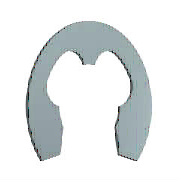
# Autodesk Inventor part: JIS B 2804 E - 3
Saved by Autodesk Inventor 2017 (Build 210142000, 142)
## iProperties
Created: 2016-02-22
Part Number: JIS B 2804 E - 3
Material: Acier, doux
Description: Rondelle élastique d´arrêt
Document SubType Name: Modeling
Standard: JIS B 2804
Designer: Adrien MARY
Standard Revision: 2010
Standards Organization: JIS
Language: fr-FR
Size Designation: 3
Categories: <MemberInstance><Categories><Category DisplayName="Pièces d'arbre" InternalName="7f7aeb1f-a693-4053-b835-cee3144e0d98" Mnemonic="SHFT"><Category DisplayName="Anneaux élastiques" InternalName="413b042a-1f46-4051-a560-0e0e417af91f" Mnemonic="CLIP"><CategoryParameter DisplayName="Epaisseur" InternalName="230c7f7c-2544-4c6d-b8d5-773e831b23fa" Mnemonic="thick"/><CategoryParameter DisplayName="Diamètre de rainure" InternalName="4054b45c-161d-4ad6-befb-f30b3855ce84" Mnemonic="grvdia"/><CategoryParameter DisplayName="Largeur de rainure" InternalName="4dde6996-4bf1-443b-8317-d4f4fc6b9be0" Mnemonic="NB"/><CategoryParameter DisplayName="Diamètre d'arbe" InternalName="a433c9ab-b9eb-4798-a453-f2210a67728e" Mnemonic="shaftdia"/><Category DisplayName="Externe" InternalName="a9a2b132-a8be-48ab-9c3d-0c324a909558" Mnemonic="OUCLIP"><CategoryParameter DisplayName="Diamètre min. d'arbre" InternalName="62b77b9b-1e86-4b9a-9911-d7c0fa48fc9a" Mnemonic="shaftdiamin"/><CategoryParameter DisplayName="Diamètre extérieur" InternalName="a3599e7b-be7c-41b5-9a50-6dab253b0906" Mnemonic="outdia"/></Category></Category></Category><Category DisplayName="Type de données" InternalName="23b78d0f-2648-40c6-8793-ca6db495c9e8" Mnemonic="DATATYPE"><CategoryParameter DisplayName="AfficherNom" InternalName="05415f3d-3907-474b-a020-eb9d644f4cf3" Mnemonic="DISPLAYNAME"/><CategoryParameter DisplayName="Norme" InternalName="0c0a119c-1e12-4c84-803f-101930972f5e" Mnemonic="STANDARD"/><CategoryParameter DisplayName="Description" InternalName="13903e3d-64b1-4950-80da-f627842ea37f" Mnemonic="DESCRIPTION"/><CategoryParameter DisplayName="Désignation" InternalName="2675968c-4ce5-49e0-a4f5-552d29089031" Mnemonic="DESIGNATION"/><CategoryParameter DisplayName="Ligne par défaut" InternalName="2af9ec52-faaa-4026-b378-f9fa4afca842" Mnemonic="DEFAULTROW"/><CategoryParameter DisplayName="Nom de dossier" InternalName="3f06958e-8713-4116-9be7-ed6184ecc97b" Mnemonic="FOLDERNAME"/><CategoryParameter DisplayName="Guide révision" InternalName="45a75005-10b1-4dfc-8d6d-dfe629f0b93c" Mnemonic="REVISIONGUID"/><CategoryParameter DisplayName="NomFichier" InternalName="8b46a4cc-9585-4fed-90c3-899f57e09a73" Mnemonic="FILENAME"/><CategoryParameter DisplayName="OrgNorm" InternalName="8f5914e1-4693-403f-8ab5-d37768198c9d" Mnemonic="STDSORG"/><CategoryParameter DisplayName="Version de la famille" InternalName="914462f6-6e19-4b14-ba84-155b9680b1d0" Mnemonic="FAMILYREVISION"/><CategoryParameter DisplayName="Version standard" InternalName="91d5a463-65c2-4fde-b823-3b7fea5e8e17" Mnemonic="STANDARDREVISION"/><CategoryParameter DisplayName="Révision de membre" InternalName="a65d44b9-392f-4f4f-857b-e4b3d54996fe" Mnemonic="MEMBERREVISION"/><CategoryParameter DisplayName="DélimiterFormat" InternalName="bc51e27b-3422-4e78-93ef-cec197ddf230" Mnemonic="CLIPFORMAT"/><CategoryParameter DisplayName="Fabricant" InternalName="cd6c7a72-a28a-4e50-99a9-2c7f4e13e5ad" Mnemonic="MANUFACTURER"/><CategoryParameter DisplayName="NomInterne" InternalName="cf1d0246-76d9-4b4a-8305-fa0409afb5c1" Mnemonic="INTERNALNAME"/><CategoryParameter DisplayName="Métrique" InternalName="e2385c5b-1ea4-4823-96a8-8de651266ec3" Mnemonic="ISMETRIC"/><Category DisplayName="Pièce" InternalName="c0e0b642-3bcb-4cc8-9e80-f96d35c4afa4" Mnemonic="PART"><CategoryParameter DisplayName="Numéro de pièce" InternalName="016b6077-bfbe-49bd-92c9-d8d59c39c941" Mnemonic="PARTNUMBER"/><CategoryParameter DisplayName="Numéro de stock" InternalName="4dba7c1c-e26c-444e-836c-b08b433409a8" Mnemonic="STOCKNUMBER"/><CategoryParameter DisplayName="Clé matière" InternalName="5c9a8adb-dd2b-4535-b97f-0a94a95fe41f" Mnemonic="MATERIALKEY"/><CategoryParameter DisplayName="Matière" InternalName="818a152a-d3c3-49ca-80ee-df7d91421b8e" Mnemonic="MATERIAL"/></Category></Category><Category DisplayName="CarteHéritée" InternalName="cd87c42b-3e48-431e-b5c0-1cbeb14dfe77" Mnemonic="LEGACYMAP"><CategoryParameter DisplayName="ID membre DA unique" InternalName="0918ad47-427f-4fed-ae26-24c81c58f590" Mnemonic="DACOOKIE"/><CategoryParameter DisplayName="ID de fusion11" InternalName="0ee8fb18-e2ed-4f39-96f6-1f4b5f50aa71" Mnemonic="MERGE11"/><CategoryParameter DisplayName="ID membre CC unique" InternalName="5193edd4-b2b0-4ab4-9d54-de900eee34e0" Mnemonic="CCCOOKIE"/><CategoryParameter DisplayName="ID de division" InternalName="72b5c83c-be7f-45c4-ae51-9160ea6deb26" Mnemonic="SPLIT"/><CategoryParameter DisplayName="IDMembre" InternalName="8e5e0294-fc51-4c8f-b3d7-003dc5ed94f6" Mnemonic="MEMBERID"/><CategoryParameter DisplayName="NomCatologue" InternalName="d99d1e27-aa94-4de2-af4c-c348882a6f4f" Mnemonic="CATALOGNAME"/><CategoryParameter DisplayName="NuméroFamille" InternalName="e705e1f4-09cb-413e-91f9-551b4188271e" Mnemonic="FAMILYNUMBER"/></Category></Categories><FamilyTemplate Id="si0132"><FamilyTemplateParameters><FamilyTemplateParameter ObjectType="kUserParameterObject" ValueType="xs:double" Id="1" ObjectReferenceKey="WDMIN"/><FamilyTemplateParameter ObjectType="kUserParameterObject" ValueType="xs:double" Id="2" ObjectReferenceKey="SNB"/><FamilyTemplateParameter ObjectType="kUserParameterObject" ValueType="xs:double" Id="3" ObjectReferenceKey="SD2"/><FamilyTemplateParameter ObjectType="kUserParameterObject" ValueType="xs:double" Id="4" ObjectReferenceKey="SD"/><FamilyTemplateParameter ObjectType="kUserParameterObject" ValueType="xs:double" Id="5" ObjectReferenceKey="ND"/><FamilyTemplateParameter ObjectType="kUserParameterObject" ValueType="xs:double" Id="6" ObjectReferenceKey="WDMAX"/><FamilyTemplateParameter ObjectType="kUserParameterObject" ValueType="xs:double" Id="7" ObjectReferenceKey="BUBRMI"/><FamilyTemplateParameter ObjectType="kUserParameterObject" ValueType="xs:double" Id="8" ObjectReferenceKey="WD"/><FamilyTemplateParameter ObjectType="kUserParameterObject" ValueType="xs:double" Id="9" ObjectReferenceKey="NND"/><FamilyTemplateParameter ObjectType="kPropertyObject" ValueType="xs:string" Id="100" ObjectReferenceKey="{32853F0F-3444-11d1-9E93-0060B03C1CA6}" SubObjectId="52"/><FamilyTemplateParameter ObjectType="kPropertyObject" ValueType="xs:string" Id="105" ObjectReferenceKey="{32853F0F-3444-11d1-9E93-0060B03C1CA6}" SubObjectId="5"/><FamilyTemplateParameter ObjectType="kPartComponentDefinitionObject" ValueType="xs:string" Id="110" SubObjectId="Material"/></FamilyTemplateParameters></FamilyTemplate><CategoryParameterMap><ParamToTemplateMap><ParamToTemplate CategoryParameter="//CategoryParameter[@InternalName='05415f3d-3907-474b-a020-eb9d644f4cf3']" ConstantValue="JIS B 2804 E"/><ParamToTemplate CategoryParameter="//CategoryParameter[@InternalName='cf1d0246-76d9-4b4a-8305-fa0409afb5c1']" ConstantValue="B983131E-6E8A-4140-85C7-FDB04EB2BDA0"/><ParamToTemplate CategoryParameter="//CategoryParameter[@InternalName='3f06958e-8713-4116-9be7-ed6184ecc97b']" ConstantValue="JIS B 2804 E"/><ParamToTemplate CategoryParameter="//CategoryParameter[@InternalName='914462f6-6e19-4b14-ba84-155b9680b1d0']" ConstantValue="10"/><ParamToTemplate CategoryParameter="//CategoryParameter[@InternalName='bc51e27b-3422-4e78-93ef-cec197ddf230']" ConstantValue="CF_INVENTOR.STDPARTS"/><ParamToTemplate CategoryParameter="//CategoryParameter[@InternalName='e2385c5b-1ea4-4823-96a8-8de651266ec3']" ConstantValue="true"/><ParamToTemplate CategoryParameter="//CategoryParameter[@InternalName='13903e3d-64b1-4950-80da-f627842ea37f']" ConstantValue="Spring Retaining Ring"/><ParamToTemplate CategoryParameter="//CategoryParameter[@InternalName='8f5914e1-4693-403f-8ab5-d37768198c9d']" ConstantValue="JIS"/><ParamToTemplate CategoryParameter="//CategoryParameter[@InternalName='0c0a119c-1e12-4c84-803f-101930972f5e']" ConstantValue="JIS B 2804"/><ParamToTemplate CategoryParameter="//CategoryParameter[@InternalName='cd6c7a72-a28a-4e50-99a9-2c7f4e13e5ad']" TemplateParameter="104"/><ParamToTemplate CategoryParameter="//CategoryParameter[@InternalName='91d5a463-65c2-4fde-b823-3b7fea5e8e17']" ConstantValue="2010"/><ParamToTemplate CategoryParameter="//CategoryParameter[@InternalName='45a75005-10b1-4dfc-8d6d-dfe629f0b93c']" ConstantValue="5afb411f-584a-4d28-a564-0e5354a33203"/><ParamToTemplate CategoryParameter="//CategoryParameter[@InternalName='2af9ec52-faaa-4026-b378-f9fa4afca842']" ConstantValue="10"/><ParamToTemplate CategoryParameter="//CategoryParameter[@InternalName='d99d1e27-aa94-4de2-af4c-c348882a6f4f']" ConstantValue="JIS"/><ParamToTemplate CategoryParameter="//CategoryParameter[@InternalName='e705e1f4-09cb-413e-91f9-551b4188271e']" ConstantValue="216"/><ParamToTemplate CategoryParameter="//CategoryParameter[@InternalName='8b46a4cc-9585-4fed-90c3-899f57e09a73']" ConstantValue="JIS B 2804 E - 3 - 5"/><ParamToTemplate CategoryParameter="//CategoryParameter[@InternalName='a65d44b9-392f-4f4f-857b-e4b3d54996fe']" ConstantValue="951B112C-607C-45C7-8E1B-EACF44DB36DB"/><ParamToTemplate CategoryParameter="//CategoryParameter[@InternalName='8e5e0294-fc51-4c8f-b3d7-003dc5ed94f6']" ConstantValue="120"/><ParamToTemplate CategoryParameter="//CategoryParameter[@InternalName='2675968c-4ce5-49e0-a4f5-552d29089031']" TemplateParameter="100"/><ParamToTemplate CategoryParameter="//CategoryParameter[@InternalName='818a152a-d3c3-49ca-80ee-df7d91421b8e']" TemplateParameter="110"/><ParamToTemplate CategoryParameter="//CategoryParameter[@InternalName='4054b45c-161d-4ad6-befb-f30b3855ce84']" TemplateParameter="5"/><ParamToTemplate CategoryParameter="//CategoryParameter[@InternalName='8bbe3f8e-44cf-40a9-a251-3a6edc8168d6']" TemplateParameter="9"/><ParamToTemplate CategoryParameter="//CategoryParameter[@InternalName='016b6077-bfbe-49bd-92c9-d8d59c39c941']" TemplateParameter="105"/><ParamToTemplate CategoryParameter="//CategoryParameter[@InternalName='230c7f7c-2544-4c6d-b8d5-773e831b23fa']" TemplateParameter="4"/><ParamToTemplate CategoryParameter="//CategoryParameter[@InternalName='4dde6996-4bf1-443b-8317-d4f4fc6b9be0']" TemplateParameter="2"/><ParamToTemplate CategoryParameter="//CategoryParameter[@InternalName='a433c9ab-b9eb-4798-a453-f2210a67728e']" TemplateParameter="8"/><ParamToTemplate CategoryParameter="//CategoryParameter[@InternalName='62b77b9b-1e86-4b9a-9911-d7c0fa48fc9a']" TemplateParameter="1"/></ParamToTemplateMap></CategoryParameterMap></MemberInstance>
Density: 7.85 g/cm^3
Appearance: Semi-poli
IsCustomPart: 0
Author: Adrien MARY
Autodesk Inventor part; units mm, degrees
ref_plane "YZ Plane" through (0, 0, 0) normal (1, 0, 0) x (0, 1, 0)
ref_plane "XZ Plane" through (0, 0, 0) normal (0, 1, 0) x (-1, 0, 0)
sketch "Esquisse1" plane through (0, 0, 0) normal (0, 0, 1) x (1, 0, 0)
  circle A0 centre (0, -2.4764) radius 2.5 construction
  line L0 (-0.3, 0.0236) -> (0, 0.0236) construction
  line L1 (-3.206, 0) -> (3.4858, 0) projected
  line L2 (-1.3748, -3.0764) -> (1.3748, -3.0764) construction
  arc A1 (-1.4207, -1.9952) -> (-1.3748, -3.0764) centre (0, -2.4764) ccw
  line L3 (0, 1.949) -> (0, -3.4788) projected
  arc A2 (-0.3, -0.6764) -> (0.3, -0.6764) centre (0, -0.6764) ccw
  arc A3 (2.6558, -4.756) -> (-2.6558, -4.756) centre (0, -2.4764) ccw
  line L4 (-1.8, -1.8764) -> (-1.506, -1.8764)
  line L5 (-0.3, -0.6764) -> (-0.3, -0.3849)
  arc A4 (-0.6, -0.1526) -> (-2.1176, -1.3469) centre (0, -2.4764) ccw
  arc A5 (-0.3, -0.3849) -> (-0.6, -0.1526) centre (-0.54, -0.3849) ccw
  arc A6 (-2.1176, -1.3469) -> (-1.8, -1.8764) centre (-1.8, -1.5164) ccw
  arc A7 (-1.4207, -1.9952) -> (-1.506, -1.8764) centre (-1.506, -1.9664) ccw
  line L6 (0, 1.0236) -> (2.5298, 1.0236) construction
  line L7 (-1.3748, -3.0764) -> (-1.8877, -4.606)
  arc A8 (-2.6558, -4.756) -> (-1.8877, -4.606) centre (-2.3143, -4.4629) ccw
  line L8 (0, -0.9764) -> (-1.2778, -0.9764) construction
  line L9 (1.3748, -3.0764) -> (1.8877, -4.606)
  arc A9 (1.8877, -4.606) -> (2.6558, -4.756) centre (2.3143, -4.4629) ccw
  arc A10 (1.3748, -3.0764) -> (1.4207, -1.9952) centre (0, -2.4764) ccw
  line L10 (1.8, -1.8764) -> (1.506, -1.8764)
  line L11 (0.3, -0.6764) -> (0.3, -0.3849)
  arc A11 (2.1176, -1.3469) -> (0.6, -0.1526) centre (0, -2.4764) ccw
  arc A12 (0.6, -0.1526) -> (0.3, -0.3849) centre (0.54, -0.3849) ccw
  arc A13 (1.8, -1.8764) -> (2.1176, -1.3469) centre (1.8, -1.5164) ccw
  arc A14 (1.506, -1.8764) -> (1.4207, -1.9952) centre (1.506, -1.9664) ccw
  point P0 (0.3, 0.0236)
  dimension "d0" = 5
  dimension "d3" = 0.6
  dimension "d4" = 0.3
  dimension "d5" = 7
  dimension "d8" = 2.4
  dimension "d9" = 0.6
  dimension "d10" = 0.24
  dimension "d11" = 0.36
  dimension "d12" = 0.09
  dimension "d13" = 0.45
  dimension "d14" = 1.5
  dimension "d15" = 1.5
  constraints: 30 point on circle, 20 end point, 15 centre point, 13 symmetric about line, 12 tangent, 8 point on line, 4 parallel, 2 coincident, 2 horizontal, 1 concentric, 1 perpendicular, 1 vertical alignment, 9 other
  measures "d0" diameter of A0
  measures "d3" distance from line of A1.centre L2
  measures "d4" radius of A2
  measures "d5" diameter of A3
  measures "d8" radius of A4
  measures "d9" distance from line of A1.centre L4
  measures "d10" radius of A5
  measures "d11" radius of A6
  measures "d12" radius of A7
  measures "d13" radius of A8
  measures "d14" distance from line of A1.centre L8
  measures "d15" radius of A1
extrude "Corps" add sketch "Esquisse1" along normal blind 0.6
ref_plane "Work Plane1" through (0, -2.4764, 0) normal (-1, 0, 0) x (0, 0, 1)
equation "\"d0\" = WD"
equation "\"d3\" = 0.2 * NND"
equation "\"d4\" = 0.1 * NND"
equation "\"d5\" = SD2"
equation "\"d8\" = 0.8 * NND"
equation "\"d9\" = 0.2 * NND"
equation "\"d10\" = 0.08 * NND"
equation "\"d11\" = 0.12 * NND"
equation "\"d12\" = 0.03 * NND"
equation "\"d13\" = 0.15 * NND"
equation "\"d14\" = 0.5 * NND"
equation "\"d15\" = 0.5 * NND"
equation "\"d16\" = SD"
equation "\"ND\" = 3.05"
equation "\"SD\" = 0.6"
equation "\"WD\" = 5"
equation "\"d1\" = 1.6 * NND"
equation "\"d2\" = NND"
equation "\"SD2\" = 7"
equation "\"d6\" = NND"
equation "\"d7\" = 0.15 * NND"
equation "\"NND\" = 3"
equation "\"WDMIN\" = 4"
equation "\"SNB\" = 0.7"
equation "\"WDMAX\" = 5"
equation "\"BUBRMI\" = 1"
body "Solid1"
